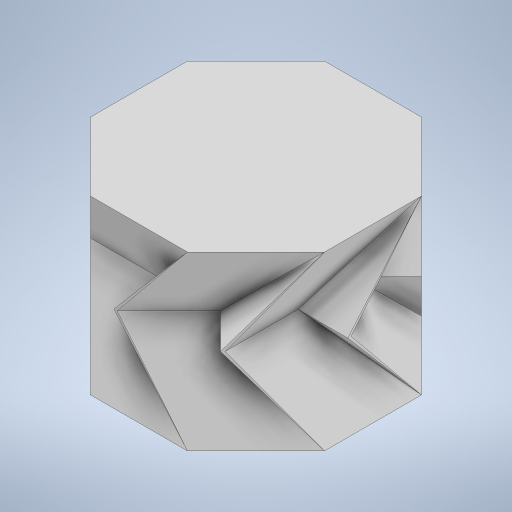
# Autodesk Inventor part: 팔각형 OV-PAM 층 한개
Saved by Autodesk Inventor 2024 (Build 280153000, 153)
## iProperties
Created: 2023-06-16
Part Number: 팔각형 OV-PAM 층 한개
Material: 일반
Document SubType Name: Modeling
Designer: jsw
Density: 1 g/cm^3
Appearance: 기본값
Mass: 15.1495 g
Surface Area: 53.0283 cm^2
Volume: 15.1495 cm^3
Author: jsw
Autodesk Inventor part; units mm, degrees
ref_plane "YZ Plane" through (0, 0, 0) normal (1, 0, 0) x (0, 1, 0)
ref_plane "XZ Plane" through (0, 0, 0) normal (0, 1, 0) x (-1, 0, 0)
sketch "스케치1" plane through (0, 0, 0) normal (0, 1, 0) x (-1, 0, 0)
  line L0 (-15.6959, 6.5015) -> (-6.5015, 15.6959)
  line L1 (-6.5015, 15.6959) -> (6.5015, 15.6959)
  line L2 (6.5015, 15.6959) -> (15.6959, 6.5015)
  line L3 (15.6959, 6.5015) -> (15.6959, -6.5015)
  line L4 (15.6959, -6.5015) -> (6.5015, -15.6959)
  line L5 (6.5015, -15.6959) -> (-6.5015, -15.6959)
  line L6 (-6.5015, -15.6959) -> (-15.6959, -6.5015)
  line L7 (-15.6959, -6.5015) -> (-15.6959, 6.5015)
  line L8 (-6.75, 16.2959) -> (6.75, 16.2959)
  line L9 (6.75, 16.2959) -> (16.2959, 6.75)
  line L10 (16.2959, 6.75) -> (16.2959, -6.75)
  line L11 (16.2959, -6.75) -> (6.75, -16.2959)
  line L12 (6.75, -16.2959) -> (-6.75, -16.2959)
  line L13 (-6.75, -16.2959) -> (-16.2959, -6.75)
  line L14 (-16.2959, -6.75) -> (-16.2959, 6.75)
  line L15 (-16.2959, 6.75) -> (-6.75, 16.2959)
  point P0 (0, 0)
  point P1 (0, 0)
  point P2 (0, 0)
  dimension "d2" = 0.6
  dimension "d54" = 13.5
  constraints: 32 end point, 2 coincident, 2 horizontal, 34 other
  measures "d2" distance between parallel lines of L10 L3
  measures "d54" distance of L8.start L8.end
extrude "돌출2" add sketch "스케치1" along normal blind 12 contours L0 L1 L2 L3 L4 L5 L6 L7 | L8 L9 L10 L11 L12 L13 L14 L15
ref_plane "작업 평면2" through (16.2959, 0, 6.75) normal (-0.8660254, -0.5, 0) x (0, 0, -1)
sketch "스케치3" plane through (16.2959, 0, 6.75) normal (1, 0, 0) x (0, 0, -1)
  line L0 (0, 0) -> (0, 12) projected
  line L1 (0, 12) -> (13.5, 12) projected
  line L2 (0, 0) -> (13.5, 0)
  line L3 (13.5, 0) -> (13.5, 12)
  line L4 (13.5, 12) -> (0, 12)
  line L5 (0, 12) -> (0, 0)
  line L6 (0, 12) -> (-7.3047, 12)
  line L7 (-9.5459, 12) -> (0, 12) projected
  line L8 (0, 0) -> (-7.3047, 12)
  line L9 (13.5, 12) -> (6.75, 12)
  line L10 (3.25, 12) -> (13.5, 0)
  point P0 (6.75, 0)
  dimension "d17" = 121.33
  dimension "d53" = 3.5
  constraints: 16 end point, 6 midpoint, 2 parallel, 2 point on line, 1 horizontal, 1 perpendicular
  measures "d17" angle of L8 L2
  measures "d53" distance of L10.start point (6.75, 12)
extrude "돌출4" cut sketch "스케치3" against normal up to surface contours L8 L6 L0 | L0 L1 L10 L2 surface through (16.2959, 0, 6.75) normal (-0.8660254, -0.5, 0)
pattern_circular "원형 패턴1" count 8 over 360 about axis through (0, -10, 0) along (0, 1, 0) of "돌출4"
mirror "미러5" about plane through (0, 12, 0) normal (0, 1, 0) of "돌출2", "돌출4", "원형 패턴1"
